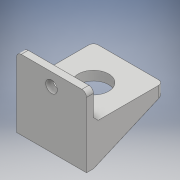
# Autodesk Inventor part: Eletronica - plug12V
Saved by Autodesk Inventor 2017 (Build 210142000, 142)
## iProperties
Created: 2020-10-25
Part Number: Eletronica - plug12V
Material: Generic
Document SubType Name: Modeling
Designer: ale
Density: 1 g/cm^3
Appearance: Default
Author: ale
Autodesk Inventor part; units mm, degrees
ref_plane "YZ Plane" through (0, 0, 0) normal (1, 0, 0) x (0, 1, 0)
ref_plane "XZ Plane" through (0, 0, 0) normal (0, 1, 0) x (-1, 0, 0)
ref_plane "XY Plane" through (0, 0, 0) normal (0, 0, 1) x (1, 0, 0)
sketch "Sketch1" plane through (0, 0, 0) normal (0, 0, 1) x (1, 0, 0)
  line L0 (-15, 15) -> (15, 15)
  line L1 (15, 15) -> (15, -15)
  line L2 (15, -15) -> (-15, -15)
  line L3 (-15, -15) -> (-15, 15)
  line L4 (-15, 15) -> (15, -15) construction
  line L5 (15, 15) -> (-15, -15) construction
  circle A0 centre (0, 0) radius 6.5
  dimension "d0" = 30
  dimension "d1" = 30
  dimension "d2" = 13
  constraints: 12 end point, 2 midpoint, 2 parallel, 1 centre point, 1 coincident, 1 horizontal, 1 perpendicular
  measures "d0" distance of L1.end L2.end
  measures "d1" distance of L0.end L1.end
  measures "d2" diameter of A0
extrude "Extrusion1" add sketch "Sketch1" along normal blind 4
sketch "Sketch2" plane through (-15, -15, 0) normal (0, -1, 0) x (1, 0, 0)
  line L0 (0, 17) -> (30, 17)
  line L1 (30, 17) -> (30, -13)
  line L2 (30, -13) -> (0, -13)
  line L3 (0, -13) -> (0, 17)
  line L4 (0, 17) -> (30, -13) construction
  line L5 (30, 17) -> (0, -13) construction
  point P0 (15, 0)
  point P1 (15, 2)
  dimension "d5" = 30
  dimension "d6" = 30
  constraints: 12 end point, 2 midpoint, 2 parallel, 1 horizontal, 1 perpendicular
  measures "d5" distance of L1.end L2.end
  measures "d6" distance of L0.end L1.end
extrude "Extrusion2" add sketch "Sketch2" along normal blind 3
ref_plane "Work Plane1" through (0, 15, 4) normal (1, 0, 0) x (0, 0, -1)
sketch "Sketch3" plane through (15, 15, 4) normal (1, 0, 0) x (0, 0, -1)
  line L0 (-13, -33) -> (17, -33) projected
  line L1 (0.0291, -33) -> (0.0291, 0)
  line L2 (4, 0) -> (4, -30) projected
  line L3 (0.0291, 0) -> (4, 0)
  line L4 (4, -30) -> (17, -30) projected
  line L5 (4, 0) -> (17, -30)
  line L6 (17, -30) -> (17, -33) projected
  line L7 (17, -30) -> (17, -33)
  line L8 (17, -33) -> (0.0291, -33)
  point P0 (4, -15)
  constraints: 10 end point, 2 perpendicular, 1 parallel, 1 point on line, 1 vertical
extrude "Extrusion3" add sketch "Sketch3" against normal blind 3 contours L4 L2 L5
mirror "Mirror1" about plane through (0, 15, 4) normal (1, 0, 0) of "Extrusion3"
chamfer "Chamfer1" distance 2 angle 45 1 edges at (0, -15, 4)
sketch "Sketch4" plane through (-15, -15, 0) normal (0, 1, 0) x (1, 0, 0)
  line L0 (0, -17) -> (30, -17) projected
  line L1 (0, -6) -> (0, -17) projected
  point P0 (15, 0)
  point P1 (15, -11.5)
  dimension "d15" = 5.5
  dimension "d16" = 15
  measures "d15" distance from line of point (15, -11.5) L0
  measures "d16" distance from line of L1 point (15, -11.5)
hole "Hole1" at (0, -15, 11.5) direction (0, -1, 0) diameter 5 end through all
fillet "Fillet1" radius 2 4 edges at (-15, 15, 2) (15, 15, 2) (15, -16.5, 17) (-15, -16.5, 17)
body "Solid1"
